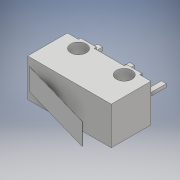
# Autodesk Inventor part: EndSwitch
Saved by Autodesk Inventor 2018 (Build 220112000, 112)
## iProperties
Created: 2020-05-13
Part Number: EndSwitch
Material: Generic
Document SubType Name: Modeling
Designer: Ivan
Density: 1 g/cm^3
Appearance: Default
Author: Ivan
Autodesk Inventor part; units mm, degrees
ref_plane "YZ Plane" through (0, 0, 0) normal (1, 0, 0) x (0, 1, 0)
ref_plane "XZ Plane" through (0, 0, 0) normal (0, 1, 0) x (-1, 0, 0)
sketch "Sketch1" plane through (0, 0, 0) normal (0, 0, 1) x (1, 0, 0)
  line L0 (6.415, 3.05) -> (6.415, -3.05)
  line L1 (6.415, -3.05) -> (-6.415, -3.05)
  line L2 (-6.415, -3.05) -> (-6.415, 3.05)
  line L3 (-4.712, 3.05) -> (-4.712, 3.4)
  line L4 (-4.712, 3.4) -> (-2.312, 3.4)
  line L5 (-2.312, 3.4) -> (-2.312, 3.05)
  line L6 (-6.415, 3.05) -> (-4.712, 3.05)
  line L7 (0, -4.34) -> (0, 4.69) construction
  line L8 (4.712, 3.05) -> (4.712, 3.4)
  line L9 (4.712, 3.4) -> (2.312, 3.4)
  line L10 (2.312, 3.4) -> (2.312, 3.05)
  line L11 (-2.312, 3.05) -> (2.312, 3.05)
  line L12 (4.712, 3.05) -> (6.415, 3.05)
  point P0 (0, 0)
  point P1 (0, 3.05)
  point P2 (6.415, 0)
  dimension "d0" = 12.83
  dimension "d1" = 6.1
  dimension "d4" = 0.35
  dimension "d5" = 2.4
  constraints: 24 end point, 7 perpendicular, 4 parallel, 4 symmetric about line, 3 horizontal, 2 midpoint, 1 horizontal alignment, 1 vertical, 1 vertical alignment
  measures "d0" distance of L0.end L1.end
  measures "d1" distance of L0.start L0.end
  measures "d4" distance of L3.start L3.end
  measures "d5" distance of L3.end L4.end
extrude "Extrusion1" add sketch "Sketch1" along normal blind 5.8
sketch "Sketch2" plane through (0, 0, 5.8) normal (0, 0, 1) x (1, 0, 0)
  circle A0 centre (-3.512, 1.85) radius 1.2
  line L0 (-2.312, 3.4) -> (-4.712, 3.4) construction
  line L1 (0, -4.34) -> (0, 4.69) construction
  line L2 (2.312, 3.05) -> (-2.312, 3.05) projected
  circle A1 centre (3.512, 1.85) radius 1.2
  line L3 (-4.712, 3.4) -> (-4.712, 3.05) projected
  line L4 (-2.312, 3.05) -> (-2.312, 3.4) projected
  point P0 (0, 0)
  point P1 (-3.512, 3.4)
  constraints: 3 tangent, 2 centre point, 1 midpoint, 1 symmetric about line, 1 vertical alignment, 1 other
extrude "Extrusion2" cut sketch "Sketch2" against normal through all
sketch "Sketch3" plane through (-2.312, 3.05, 0) normal (0, 1, 0) x (1, 0, 0)
  line L0 (6.827, -2.65) -> (7.577, -2.65)
  line L1 (7.577, -2.65) -> (7.577, -3.15)
  line L2 (7.577, -3.15) -> (6.827, -3.15)
  line L3 (6.827, -3.15) -> (6.827, -2.65)
  line L4 (8.727, 0) -> (7.024, 0) construction
  line L5 (8.727, 0) -> (8.727, -5.8) construction
  line L6 (-2.203, -2.65) -> (-2.953, -2.65)
  line L7 (-2.953, -2.65) -> (-2.953, -3.15)
  line L8 (-2.953, -3.15) -> (-2.203, -3.15)
  line L9 (-2.203, -3.15) -> (-2.203, -2.65)
  line L10 (1.937, -2.65) -> (2.687, -2.65)
  line L11 (2.687, -2.65) -> (2.687, -3.15)
  line L12 (2.687, -3.15) -> (1.937, -3.15)
  line L13 (1.937, -3.15) -> (1.937, -2.65)
  line L14 (-6.669, 0) -> (11.293, 0) construction
  line L15 (-4.103, 0) -> (-4.103, -5.8) projected
  line L16 (-4.103, -2.9) -> (8.727, -2.9) construction
  line L17 (2.312, 0) -> (2.312, -5.8) construction
  line L18 (-4.103, -5.8) -> (8.727, -5.8) construction
  point P0 (7.577, -2.9)
  point P1 (2.687, -2.9)
  point P2 (2.312, -2.9)
  point P3 (2.312, -2.9)
  point P4 (-2.953, -2.9)
  point P5 (2.312, -2.65)
  dimension "d10" = 0.75
  dimension "d11" = 0.5
  dimension "d12" = 1.15
  constraints: 28 end point, 9 midpoint, 4 parallel, 3 horizontal alignment, 2 equal length, 2 horizontal, 2 perpendicular, 1 vertical alignment
  measures "d10" distance of L1.end L2.end
  measures "d11" distance of L0.end L1.end
  measures "d12" distance between parallel lines of L5 L1
extrude "Extrusion3" add sketch "Sketch3" along normal blind 3.5
ref_plane "Work Plane1" through (0, 0, 2.9) normal (0, 0, 1) x (1, 0, 0)
sketch "Sketch5" plane through (0, 0, 2.9) normal (0, 0, 1) x (1, 0, 0)
  line L0 (-6.415, -3.05) -> (6.415, -3.05) construction
  line L1 (-6.1061, -3.05) -> (5.2368, -6.3025)
  line L2 (-6.1061, -3.05) -> (5.6939, -3.05) construction
  line L3 (5.2368, -6.3025) -> (5.223, -6.3506)
  line L4 (5.2368, -6.3025) -> (5.2868, -6.3025) construction
  line L5 (5.223, -6.3506) -> (-6.1199, -3.0981)
  line L6 (-6.1061, -3.05) -> (-6.1199, -3.0981)
  point P0 (0, 0)
  dimension "d17" = 11.8
  dimension "d18" = 16
  dimension "d19" = 0.05
  dimension "d20" = 106
  dimension "d21" = 11.8
  constraints: 12 end point, 2 equal length, 2 horizontal, 2 perpendicular, 1 point on line
  measures "d17" distance of L1.start L1.end
  measures "d18" angle of L1 L2
  measures "d19" distance of L1.end L3.end
  measures "d20" angle of L3 L4
  measures "d21" distance of L3.end L5.end
extrude "Extrusion4" add sketch "Sketch5" along normal mid plane 3.3
body "Solid1"
